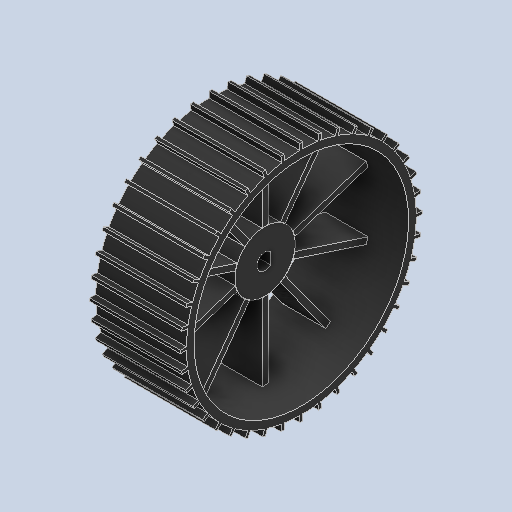
# Autodesk Inventor part: Roue
Saved by Autodesk Inventor 2026.2 (Build 302298010, 298A)
## iProperties
Created: 2026-03-30
Part Number: Roue
Material: Générique
Document SubType Name: Modeling
Designer: Genon
Density: 1 g/cm^3
Appearance: Caoutchouc - Noir
Author: Genon
Autodesk Inventor part; units mm, degrees
ref_plane "YZ Plane" through (0, 0, 0) normal (1, 0, 0) x (0, 1, 0)
ref_plane "XY Plane" through (0, 0, 0) normal (0, 0, 1) x (1, 0, 0)
sketch "Esquisse1" plane through (0, 0, 0) normal (0, 0, 1) x (1, 0, 0)
  line L0 (0, 0) -> (0, 38)
  line L1 (0, 38) -> (30, 38)
  line L2 (30, 38) -> (30, 35.5)
  line L3 (30, 35.5) -> (0, 35.5)
  line L4 (0, 0) -> (0, 10)
  line L5 (0, 10) -> (18, 10)
  line L6 (18, 10) -> (18, 0)
  line L7 (18, 0) -> (0, 0)
  line L8 (-6, 0) -> (36, 0) projected
  dimension "d0" = 38
  dimension "d1" = 30
  dimension "d2" = 2.5
  dimension "d3" = 10
  dimension "d4" = 18
  constraints: 16 end point, 6 perpendicular, 2 point on line, 1 vertical
  measures "d0" distance of L0.start L0.end
  measures "d1" distance of L0.end L1.end
  measures "d2" distance of L1.end L2.end
  measures "d3" distance of L0.start L4.end
  measures "d4" distance of L4.end L5.end
sketch "Esquisse1 outline for Révolution1" plane through (0, 0, 0) normal (0, 0, 1) x (1, 0, 0)
  line L0 (0, 0) -> (18, 0)
  line L1 (0, 10) -> (0, 0)
  line L2 (18, 10) -> (0, 10)
  line L3 (18, 0) -> (18, 10)
  line L4 (30, 35.5) -> (30, 38)
  line L5 (0, 35.5) -> (30, 35.5)
  line L6 (0, 38) -> (0, 35.5)
  line L7 (30, 38) -> (0, 38)
revolve "Révolution1" add sketch "Esquisse1 outline for Révolution1" angle 360 about axis through (-10, 0, 0) along (1, 0, 0)
ref_plane "Plan de construction1" through (0, 10, 0) normal (0, 1, 0) x (-1, 0, 0)
sketch "Esquisse2" plane through (0, 10, 0) normal (0, 1, 0) x (-1, 0, 0)
  line L0 (0, 0) -> (0, 1)
  line L1 (0, 38) -> (0, -38) projected
  line L2 (0, 1) -> (-18, 1)
  line L3 (-18, 1) -> (-18, -1)
  line L4 (-18, -1) -> (0, -1)
  line L5 (0, 0) -> (0, -1)
  dimension "d7" = 1
  dimension "d8" = 18
  dimension "d9" = 2
  dimension "d10" = 90
  constraints: 10 end point, 3 perpendicular, 2 point on line, 1 collinear
  measures "d7" distance of L0.start L0.end
  measures "d8" distance of L0.end L2.end
  measures "d9" distance of L2.end L3.end
  measures "d10" angle of L3 L2
sketch "Esquisse2 outline for Extrusion1" plane through (0, 10, 0) normal (0, 1, 0) x (-1, 0, 0)
  line L0 (-18, 1) -> (-18, -1)
  line L1 (0, 1) -> (-18, 1)
  line L2 (0, 0) -> (0, 1)
  line L3 (0, -1) -> (0, 0)
  line L4 (-18, -1) -> (0, -1)
extrude "Extrusion1" add sketch "Esquisse2 outline for Extrusion1" along normal up to surface
sketch "Esquisse3" plane through (30, 0, 0) normal (1, 0, 0) x (0, 0, -1)
  circle A0 centre (0, 0) radius 38
  circle A1 centre (0, 0) radius 38
  line L0 (0, 38) -> (0, 40)
  line L1 (0, 40) -> (0.5, 40)
  line L2 (0.5, 40) -> (0.5, 37.99671)
  line L3 (0, 40) -> (-0.5, 40)
  line L4 (-0.5, 40) -> (-0.5, 37.99671)
  dimension "d13" = 2
  dimension "d14" = 0.5
  dimension "d15" = 0.5
  constraints: 10 end point, 3 perpendicular, 3 point on circle, 1 point on line, 1 vertical
  measures "d13" distance of L0.start L0.end
  measures "d14" distance of L0.end L1.end
  measures "d15" distance of L0.end L3.end
sketch "Esquisse3 outline for Extrusion2" plane through (30, 0, 0) normal (1, 0, 0) x (0, 0, -1)
  line L0 (0.5, 40) -> (0, 40)
  line L1 (0.5, 37.99671) -> (0.5, 40)
  arc A0 (-0.5, 37.99671) -> (0.5, 37.99671) centre (0, 0) cw
  line L2 (-0.5, 40) -> (-0.5, 37.99671)
  line L3 (0, 40) -> (-0.5, 40)
extrude "Extrusion2" add sketch "Esquisse3 outline for Extrusion2" against normal blind 30
pattern_circular "Réseau circulaire1" count 10 over 360 about axis through (9, 0, 0) along (1, 0, 0) of "Extrusion1"
pattern_circular "Réseau circulaire2" count 40 over 360 about axis through (9, 0, 0) along (1, 0, 0) of "Extrusion2"
sketch "Esquisse4" plane through (0, 0, 0) normal (-1, 0, 0) x (0, 0, 1)
  circle A0 centre (0, 0) radius 2.65
  circle A1 centre (0, 0) radius 2.85
  line L0 (2.85, 0) -> (-1.8, 0)
  line L1 (-1.8, 0) -> (-1.8, 2.209638)
  line L2 (-1.8, 0) -> (-1.8, -2.209638)
  point P0 (-1.8, -1.944865)
  point P1 (-1.8, 1.944865)
  dimension "d24" = 5.3
  dimension "d25" = 5.7
  dimension "d26" = 4.65
  constraints: 6 end point, 3 point on circle, 2 centre point, 2 coincident, 1 horizontal, 1 perpendicular, 1 point on line
  measures "d24" diameter of A0
  measures "d25" diameter of A1
  measures "d26" distance of L0.start L0.end
sketch "Esquisse4 outline for Extrusion3" plane through (0, 0, 0) normal (-1, 0, 0) x (0, 0, 1)
  line L0 (-1.8, 0) -> (-1.8, -1.944865)
  line L1 (-1.8, 1.944865) -> (-1.8, 0)
  arc A0 (-1.8, -1.944865) -> (-1.8, 1.944865) centre (0, 0) ccw
extrude "Extrusion3" cut sketch "Esquisse4 outline for Extrusion3" against normal blind 25
sketch "Esquisse7" plane through (0, 0, 0) normal (-1, 0, 0) x (0, 0, 1)
  circle A0 centre (0, 0) radius 2.65
  dimension "d30" = 5.3
  constraints: 1 centre point, 1 coincident
  measures "d30" diameter of A0
sketch "Esquisse7 outline for Extrusion4" plane through (0, 0, 0) normal (-1, 0, 0) x (0, 0, 1)
  circle A0 centre (0, 0) radius 2.65
extrude "Extrusion4" cut sketch "Esquisse7 outline for Extrusion4" against normal blind 7
sketch "Esquisse8" plane through (0, 0, 0) normal (-1, 0, 0) x (0, 0, 1)
  arc A0 (-1.8, 1.944865) -> (-1.8, -1.944865) centre (0, 0) ccw
  circle A1 centre (0, 0) radius 35.5
  line L0 (-1.8, 1.944865) -> (-1.8, -1.944865)
  arc A2 (-1.8, 1.944865) -> (-1.8, -1.944865) centre (0, 0) ccw
  constraints: 1 centre point, 1 coincident
sketch "Esquisse8 outline for Extrusion5" plane through (0, 0, 0) normal (-1, 0, 0) x (0, 0, 1)
  circle A0 centre (0, 0) radius 35.5
extrude "Extrusion5" cut sketch "Esquisse8 outline for Extrusion5" against normal blind 4
